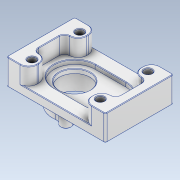
# Autodesk Inventor part: ServoMount
Saved by Autodesk Inventor 2020 (Build 240168000, 168)
## iProperties
Created: 2019-12-15
Part Number: ServoMount
Material: Aluminum 6061
Document SubType Name: Modeling
Designer: Kjell
Density: 2.7 g/cm^3
Appearance: Aluminum - Flat
Author: Kjell
Autodesk Inventor part; units mm, degrees
ref_plane "YZ Plane" through (0, 0, 0) normal (1, 0, 0) x (0, 1, 0)
ref_plane "XZ Plane" through (0, 0, 0) normal (0, 1, 0) x (-1, 0, 0)
ref_plane "XY Plane" through (0, 0, 0) normal (0, 0, 1) x (1, 0, 0)
sketch "Sketch1" plane through (0, 0, 0) normal (0, 0, 1) x (1, 0, 0)
  line L0 (-20, 20) -> (38, 20)
  line L1 (38, 20) -> (38, -20)
  line L2 (38, -20) -> (-20, -20)
  line L3 (-20, -20) -> (-20, 20)
  line L4 (-20, 20) -> (38, -20) construction
  line L5 (38, 20) -> (-20, -20) construction
  circle A0 centre (0, 0) radius 9
  circle A1 centre (-11, -14) radius 2.25
  circle A2 centre (-11, 14) radius 2.25
  circle A3 centre (29, 14) radius 2.25
  circle A4 centre (29, -14) radius 2.25
  line L6 (0, 0) -> (-29.1086, 0) construction
  point P0 (9, 0)
  point P1 (9, 0)
  dimension "d0" = 58
  dimension "d1" = 40
  dimension "d2" = 20
  dimension "d3" = 18
  dimension "d4" = 4.5
  dimension "d5" = 4.5
  dimension "d6" = 4.5
  dimension "d7" = 4.5
  dimension "d8" = 40
  dimension "d9" = 11
  dimension "d28" = 28
  constraints: 14 end point, 5 centre point, 3 horizontal alignment, 3 midpoint, 2 horizontal, 2 parallel, 2 vertical alignment, 1 coincident, 1 perpendicular, 1 symmetric about line
  measures "d0" distance of L1.end L2.end
  measures "d1" distance of L0.end L1.end
  measures "d2" distance from line of point (0, 0) L3
  measures "d3" diameter of A0
  measures "d4" diameter of A1
  measures "d5" diameter of A2
  measures "d6" diameter of A3
  measures "d7" diameter of A4
  measures "d8" distance of A4.centre A1.centre
  measures "d9" horizontal distance of A1.centre point (0, 0)
  measures "d28" distance of A2.centre A1.centre
extrude "Extrusion1" add sketch "Sketch1" against normal blind 5
fillet "Fillet1" radius 1 4 edges at (-20, -20, -2.5) (38, -20, -2.5) (38, 20, -2.5) (-20, 20, -2.5)
sketch "Sketch3" plane through (0, 0, 0) normal (0, 0, 1) x (1, 0, 0)
  arc A0 (-19, 20) -> (-20, 19) centre (-19, 19) ccw projected
  line L0 (-20, 19) -> (-20, -19) projected
  arc A1 (-20, -19) -> (-19, -20) centre (-19, -19) ccw projected
  line L1 (-19, -20) -> (37, -20) projected
  arc A2 (37, -20) -> (38, -19) centre (37, -19) ccw projected
  line L2 (38, -19) -> (38, 19) projected
  arc A3 (38, 19) -> (37, 20) centre (37, 19) ccw projected
  line L3 (37, 20) -> (-19, 20) projected
  circle A4 centre (29, 14) radius 2.25 projected
  circle A5 centre (29, -14) radius 2.25 projected
  circle A6 centre (-11, -14) radius 2.25 projected
  circle A7 centre (-11, 14) radius 2.25 projected
  circle A8 centre (0, 0) radius 9 projected
  line L4 (0, 0) -> (-27.9086, 0) construction
  line L5 (-7, 9) -> (-15, 9)
  line L6 (-15, 9) -> (-15, -9)
  line L7 (-15, -9) -> (-7, -9)
  line L8 (-7, 20) -> (-7, 9)
  line L9 (-7, -9) -> (-7, -20)
  line L10 (25, 20) -> (25, -20.2635)
  line L11 (25, 9) -> (33, 9)
  line L12 (33, 9) -> (33, -9)
  line L13 (33, -9) -> (25, -9)
  line L14 (25, -9) -> (25, 9)
  point P0 (25, -20)
  dimension "d30" = 18
  dimension "d31" = 5
  dimension "d33" = 4
  dimension "d34" = 4
  dimension "d35" = 18
  dimension "d36" = 5
  constraints: 22 end point, 5 perpendicular, 4 point on line, 3 horizontal, 3 parallel, 2 other
  measures "d30" distance between parallel lines of L7 L5
  measures "d31" distance between parallel lines of L6 L0
  measures "d33" distance from line of L8 A7.centre
  measures "d34" distance from line of L10 A4.centre
  measures "d35" distance of L11.end L12.end
  measures "d36" distance between parallel lines of L2 L12
extrude "Extrusion2" add sketch "Sketch3" along normal blind 10 contours L3 L8 L5 L6 L7 L9 L1 A1 L0 A0 | L3 A3 L2 A2 L1 L10 L13 L12 L11
fillet "Fillet2" radius 5 8 edges at (-7, -20, 5) (-7, 20, 5) (25, -20, 5) (25, 20, 5) (-7, -9, 5) (25, -9, 5) (-7, 9, 5) (25, 9, 5)
fillet "Fillet2" radius 3 4 edges at (33, -9, 5) (33, 9, 5) (-15, 9, 5) (-15, -9, 5)
sketch "Sketch4" plane through (0, 0, 0) normal (0, 0, 1) x (1, 0, 0)
  circle A0 centre (0, 0) radius 9 projected
  line L0 (0, 0) -> (18, 0) construction
  line L1 (0, -12) -> (18, -12)
  line L2 (18, 12) -> (0, 12)
  arc A1 (0, 12) -> (0, -12) centre (0, 0) ccw
  arc A2 (18, -12) -> (18, 12) centre (18, 0) ccw
  point P0 (9, 0)
  dimension "d41" = 24
  dimension "d42" = 18
  constraints: 8 end point, 4 point on circle, 4 tangent, 2 centre point, 1 horizontal, 1 midpoint, 1 parallel
  measures "d41" diameter of A2
  measures "d42" distance of L0.end L0.start
extrude "Extrusion3" cut sketch "Sketch4" against normal blind 2.5
sketch "Sketch5" plane through (0, 0, -5) normal (0, 0, -1) x (-1, 0, 0)
  circle A0 centre (0, 0) radius 9 projected
  circle A1 centre (0, 0) radius 10.525
  line L0 (0, 0) -> (31.9474, 0) construction
  circle A2 centre (0, 0) radius 14 construction
  arc A3 (12.7143, -2.7105) -> (12.7143, 2.7105) centre (14, 0) ccw
  arc A4 (-4.0098, 12.3662) -> (-8.7045, 9.6556) centre (-7, 12.1244) ccw
  arc A5 (-8.7045, -9.6556) -> (-4.0098, -12.3662) centre (-7, -12.1244) ccw
  arc A6 (-4.0098, -12.3662) -> (12.7143, -2.7105) centre (0, 0) ccw
  arc A7 (12.7143, 2.7105) -> (-4.0098, 12.3662) centre (0, 0) ccw
  arc A8 (-8.7045, 9.6556) -> (-8.7045, -9.6556) centre (0, 0) ccw
  dimension "d47" = 28
  dimension "d45" = 21.05
  dimension "d48" = 6
  dimension "d51" = 360
  constraints: 12 point on circle, 7 centre point, 3 coincident, 2 end point, 1 horizontal, 1 horizontal alignment, 1 point on line, 15 other
  measures "d45" diameter of A1
  measures "d48" diameter of A3
extrude "Extrusion4" add sketch "Sketch5" along normal blind 10 contours A6 A5 A8 A4 A7 A3
fillet "Fillet3" radius 3 6 edges at (-12.7143, 2.7105, -10) (4.0098, 12.3662, -10) (-12.7143, -2.7105, -10) (4.0098, -12.3662, -10) (8.7045, -9.6556, -10) (8.7045, 9.6556, -10)
chamfer "Chamfer2" distance 0.3 angle 45 67 edges at (-15, 0, 10) (-14.1213, 8.1213, 10) (-12, 9, 10) (-8.4644, 10.4644, 10) (-7, 14.5, 10) (-8.4644, 18.5356, 10) (-15.5, 20, 10) (-19.7071, 19.7071, 10) (-20, 0, 10) (-19.7071, -19.7071, 10) (-15.5, -20, 10) (-8.4644, -18.5356, 10) (-7, -14.5, 10) (-8.4644, -10.4644, 10) (-12, -9, 10) (-14.1213, -8.1213, 10) (-13.25, -14, 10) (-13.25, 14, 10) (9, -12, 0) (-12, 0, 0) (9, 12, 0) (30, 0, 0) (-9, 0, -2.5) (26.75, -14, 10) (26.75, 14, 10) (38, 0, 10) (37.7071, 19.7071, 10) (33.4999, 20, 10) (26.4644, 18.5356, 10) (25, 14.5, 10) (26.4644, 10.4644, 10) (30, 9, 10) (32.1213, 8.1213, 10) (33, 0, 10) (32.1213, -8.1213, 10) (30, -9, 10) (26.4644, -10.4644, 10) (25, -14.5, 10) (26.4644, -18.5356, 10) (33.4999, -20, 10) (37.7071, -19.7071, 10) (9, -20, 0) (9, 20, 0) (38, 0, -5) (37.7071, -19.7071, -5) (9, -20, -5) (-19.7071, -19.7071, -5) (-20, 0, -5) (-19.7071, 19.7071, -5) (9, 20, -5) (37.7071, 19.7071, -5) (13, 0, -15) (9.6022, -9.4689, -15) (8.5, -14.7224, -15) (3.3992, -13.0502, -15) (-6.5, -11.2583, -15) (-13.0014, -3.5813, -15) (-17, 0, -15) (-13.0014, 3.5813, -15) (-6.5, 11.2583, -15) (3.3992, 13.0502, -15) (8.5, 14.7224, -15) (9.6022, 9.4689, -15) (26.75, -14, -5) (26.75, 14, -5) (-13.25, -14, -5) (-13.25, 14, -5)
sketch "Sketch2" plane through (0, 0, 0) normal (0, 0, 1) x (1, 0, 0)
  circle A0 centre (0, 0) radius 9 projected
  circle A1 centre (0, 0) radius 14 construction
  line L0 (0, 0) -> (-14.8721, 0) construction
  point P0 (-14, 0)
  point P1 (7, -12.1244)
  point P2 (7, 12.1244)
  dimension "d13" = 28
  dimension "d16" = 360
  constraints: 2 end point, 1 coincident, 1 horizontal, 1 horizontal alignment, 1 point on line, 6 other
sketch "Sketch6" plane through (0, 0, -15) normal (0, 0, -1) x (-1, 0, 0)
  point P0 (14, 0)
  point P1 (-7, -12.1244)
  point P2 (-7, 12.1244)
hole "Hole2" at (-14, 0, -15) at (7, -12.1244, -15) at (7, 12.1244, -15) direction (0, 0, 1) diameter 2.459 depth 8 tip angle 120 thread size "M3x0.5" class "6H" standard "ISO Metric profile"
body "Solid1"
